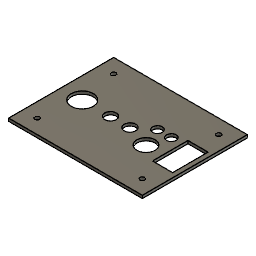
control+panel (Autodesk Fusion 360 design; units mm, degrees)
part number: 2026-03-02-18-46-18-823
Autodesk Fusion 360 part; units mm, degrees
sketch "Sketch1" plane through (0, 0, 0) normal (0, 1, 0) x (1, 0, 0)
  line L0 (-51.7543, 55.7578) -> (88.2457, 55.7578)
  line L1 (88.2457, 55.7578) -> (88.2457, -54.2422)
  line L2 (88.2457, -54.2422) -> (-51.7543, -54.2422)
  line L3 (-51.7543, -54.2422) -> (-51.7543, 55.7578)
  line L4 (-34.6167, 55.7578) -> (-34.6167, 25.7578)
  line L5 (-4.6987, -54.2422) -> (-4.6987, -24.2422)
  line L6 (-51.7543, -24.2422) -> (88.2457, -24.2422)
  line L7 (-51.7543, 25.7578) -> (88.2457, 25.7578)
  line L8 (62.4536, 19.2578) -> (83.4536, 19.2578)
  line L9 (83.4536, 19.2578) -> (83.4536, -17.7422)
  line L10 (83.4536, -17.7422) -> (62.4536, -17.7422)
  line L11 (62.4536, -17.7422) -> (62.4536, 19.2578)
  line L12 (28.1038, -13.9922) -> (12.5038, -13.9922)
  line L13 (12.5038, -13.9922) -> (12.5038, 15.5078)
  circle A0 centre (20.3038, 0.7578) radius 6
  line L14 (12.5038, -13.9922) -> (28.1038, 15.5078)
  line L15 (12.5038, 15.5078) -> (28.1038, -13.9922)
  line L16 (12.5038, 15.5078) -> (28.1038, 15.5078)
  line L17 (28.1038, 15.5078) -> (28.1038, -13.9922)
  line L18 (-7.8, 15.5078) -> (7.8, 15.5078)
  line L19 (-7.8, 15.5078) -> (7.8, -13.9922)
  circle A1 centre (0, 0.7578) radius 6
  line L20 (-7.8, -13.9922) -> (7.8, 15.5078)
  line L21 (-7.8, -13.9922) -> (-7.8, 15.5078)
  line L22 (7.8, 15.5078) -> (7.8, -13.9922)
  line L23 (7.8, -13.9922) -> (-7.8, -13.9922)
  line L24 (-51.7543, 0.7578) -> (88.2457, 0.7578)
  circle A2 centre (36.5574, 13.2578) radius 5
  line L25 (88.2457, 25.7578) -> (88.2457, 0.7578)
  line L26 (88.2457, 0.7578) -> (88.2457, -24.2422)
  line L27 (88.2457, 13.2578) -> (-51.7543, 13.2578)
  circle A3 centre (51.09, 13.2578) radius 5
  circle A4 centre (44.5885, -6.7531) radius 9.5
  circle A5 centre (-29.6042, 0.7578) radius 11.5
  point P0 (20.3038, 0.7578)
  point P1 (35.7195, -1.6286)
  point P2 (0, 0.7578)
  point P3 (-51.7543, 0.7578)
  point P4 (83.4536, 0.7578)
  point P5 (88.2457, 13.2578)
  point P6 (88.2457, -11.7422)
  dimension "d1" = 140
  dimension "d2" = 110
  dimension "d3" = 30
  dimension "d4" = 30
  dimension "d5" = 21
  dimension "d6" = 37
  dimension "d10" = 15.6
  dimension "d11" = 29.5
  dimension "d12" = 12
  dimension "d16" = 15.6
  dimension "d17" = 29.5
  dimension "d18" = 12
  dimension "d19" = 10
  dimension "d20" = 10
  dimension "d21" = 19
  dimension "d22" = 23
  constraint horizontal L0
  constraint vertical L1
  constraint horizontal L2
  constraint vertical L3
  constraint coincident L0 L4.start
  constraint perpendicular L0 L4
  constraint coincident L2 L5.start
  constraint perpendicular L2 L5
  constraint coincident L3 L6.start
  constraint coincident L1 L6.end
  constraint perpendicular L1 L6
  constraint coincident L3 L7.start
  constraint coincident L1 L7.end
  constraint perpendicular L1 L7
  constraint coincident L4.end L7
  constraint coincident L5.end L6
  constraint horizontal L8
  constraint vertical L9
  constraint horizontal L10
  constraint vertical L11
  constraint horizontal L16
  constraint vertical L17
  constraint horizontal L12
  constraint vertical L13
  constraint midpoint P0 L14
  constraint horizontal L18
  constraint vertical L22
  constraint horizontal L23
  constraint vertical L21
  constraint midpoint P2 L20
  constraint midpoint L3 P3
  constraint coincident P3 L24.start
  constraint midpoint L1 L24.end
  constraint coincident P2 L24
  constraint coincident P0 L24
  constraint midpoint L9 P4
  constraint coincident L24 P4
  constraint midpoint L25 P5
  constraint midpoint L26 P6
  constraint coincident P5 L27.start
  constraint coincident L3 L27.end
  constraint perpendicular L3 L27
  constraint coincident A2.centre L27
  constraint coincident L27 A3.centre
  constraint coincident L24 A5.centre
  measures "d1" distance of L0.start L0.end
  measures "d2" distance of L0.start L2.end
  measures "d3" distance of L4.start L4.end
  measures "d4" distance of L5.start L5.end
  measures "d5" distance of L8.start L8.end
  measures "d6" distance of L8.start L10.end
  measures "d10" distance of L13.end L14.end
  measures "d11" distance of L13.end L12.end
  measures "d12" diameter of A0
  measures "d16" distance of L18.end L18.start
  measures "d17" distance of L20.start L18.start
  measures "d18" diameter of A1
  measures "d19" diameter of A2
  measures "d20" diameter of A3
  measures "d21" diameter of A4
  measures "d22" diameter of A5
extrude "Extrude1" add sketch "Sketch1" along normal blind 3 contours L0 L3 L4 L7 | L0 L1 L4 L7 | L1 L3 L7 L8 L9 L11 L13 L16 L17 L18 L21 L22 A2 L25 L27 A3 | L3 L21 L24 L27 A5 | L1 L3 L6 L9 L10 L11 L12 L13 L17 L21 L22 L23 L24 L26 A4 A5 | L19 A1 L21 L24 L27 | L19 L21 L27 | L1 L9 L24 L25 L27 | L2 L3 L5 L6 | A1 L20 L21 L24 | L18 L19 L20 L27 | L19 A1 L20 L27 | L1 L2 L5 L6 | L19 A1 L20 L23 | L20 L22 L27 | A1 L20 L22 L24 L27 | L11 L17 L24 A2 L27 A3 A4 | L19 A1 L22 L24 | L13 L22 L24 L27 | L13 A0 L15 L24 L27 | L13 L15 L27 | L13 A0 L14 L24 | L14 L15 L16 L27 | A0 L14 L15 L27 | L12 A0 L14 L15 | L14 L17 L27 | A0 L14 L17 L24 L27 | A0 L15 L17 L24
sketch "Sketch2" plane through (0, 3, 0) normal (0, 1, 0) x (-1, 0, 0)
  line L0 (-83.4536, 17.7422) -> (-62.4536, 17.7422)
  line L1 (-62.4536, 17.7422) -> (-62.4536, -19.2578)
  line L2 (-62.4536, -19.2578) -> (-83.4536, -19.2578)
  line L3 (-83.4536, -19.2578) -> (-83.4536, 17.7422)
  circle A0 centre (-36.5574, -13.2578) radius 5
  circle A1 centre (-20.3038, -0.7578) radius 6
  circle A2 centre (-51.09, -13.2578) radius 5
  circle A3 centre (0, -0.7578) radius 6
  circle A4 centre (-44.5885, 6.7531) radius 9.5
  circle A5 centre (29.6042, -0.7578) radius 11.5
  line L4 (-88.2457, 54.2422) -> (-88.2457, -55.7578)
  line L5 (-88.2457, -55.7578) -> (51.7543, -55.7578)
  line L6 (51.7543, -55.7578) -> (51.7543, 54.2422)
  line L7 (51.7543, 54.2422) -> (-88.2457, 54.2422)
  line L8 (-17.1333, -55.7578) -> (-17.1333, -40.7578)
  line L9 (51.7543, -40.7578) -> (-88.2457, -40.7578)
  line L10 (-18.2457, 54.2422) -> (-18.2457, 39.2422)
  line L11 (51.7543, 39.2422) -> (-88.2457, 39.2422)
  line L12 (51.7543, -40.7578) -> (36.7543, -40.7578)
  line L13 (-88.2457, -40.7578) -> (-73.2457, -40.7578)
  line L14 (51.7543, 39.2422) -> (36.7543, 39.2422)
  line L15 (-88.2457, 39.2422) -> (-73.2457, 39.2422)
  point P0 (36.7543, -40.7578)
  point P1 (36.7543, 39.2422)
  point P2 (-73.2457, 39.2422)
  point P3 (-73.2457, -40.7578)
  dimension "d25" = 15
  dimension "d26" = 15
  dimension "d27" = 15
  dimension "d28" = 15
  dimension "d29" = 15
  dimension "d30" = 15
  constraint coincident L5 L8.start
  constraint perpendicular L5 L8
  constraint coincident L6 L9.start
  constraint coincident L4 L9.end
  constraint perpendicular L4 L9
  constraint midpoint L7 L10.start
  constraint perpendicular L7 L10
  constraint coincident L6 L11.start
  constraint coincident L4 L11.end
  constraint perpendicular L4 L11
  constraint perpendicular L6 L12
  constraint perpendicular L4 L13
  constraint perpendicular L6 L14
  constraint perpendicular L4 L15
  constraint coincident P0 L12.end
  constraint coincident P1 L14.end
  constraint coincident P2 L15.end
  constraint coincident P3 L13.end
  measures "d25" distance of L8.start L8.end
  measures "d26" distance of L10.start L10.end
  measures "d27" distance of L9.start P0
  measures "d28" distance of L9.end P3
  measures "d29" distance of L11.start P1
  measures "d30" distance of L11.end P2
hole "Hole1" at (-36.7543, 3, -40.7578) at (-36.7543, 3, 39.2422) at (73.2457, 3, -40.7578) at (73.2457, 3, 39.2422) direction (0, -1, 0) diameter 4.8 depth 15 tip angle 180
